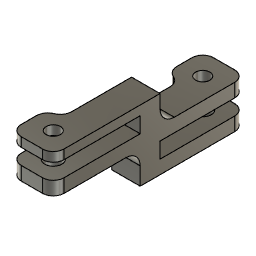
master v6 (Autodesk Fusion 360 archive; units mm, degrees)
design "Linkage"
Autodesk Fusion 360 part; units mm, degrees
sketch "Sketch1" plane through (0, 0, 0) normal (1, 0, 0) x (0, 1, 0)
  line L0 (-75.822, 4.0286) -> (-63.122, 4.0286)
  line L1 (-56.772, -1.661) -> (-41.532, -1.661)
  line L2 (-41.532, 5.959) -> (-53.8576, 5.959)
  line L3 (-60.2076, 10.8866) -> (-75.822, 10.8866)
  line L4 (-75.822, 4.0286) -> (-75.822, 6.4416)
  line L5 (-75.822, 6.4416) -> (-60.3127, 6.4416)
  line L6 (-60.3127, 6.4416) -> (-60.3127, 9.2356)
  line L7 (-60.3127, 9.2356) -> (-75.822, 9.2356)
  line L8 (-75.822, 9.2356) -> (-75.822, 10.8866)
  line L9 (-41.532, -1.661) -> (-41.532, 0.752)
  line L10 (-41.532, 0.752) -> (-56.772, 0.752)
  line L11 (-56.772, 0.752) -> (-56.772, 3.546)
  line L12 (-56.772, 3.546) -> (-41.532, 3.546)
  line L13 (-41.532, 3.546) -> (-41.532, 5.959)
  line L14 (-60.2076, 10.8866) -> (-56.772, 10.8866)
  line L15 (-56.772, 10.8866) -> (-56.772, 5.959)
  line L16 (-56.772, 5.959) -> (-53.8576, 5.959)
  line L17 (-56.772, -1.661) -> (-60.3127, -1.661)
  line L18 (-60.3127, -1.661) -> (-60.3127, 4.0286)
  line L19 (-60.3127, 4.0286) -> (-63.122, 4.0286)
  dimension "d2" = 7.62
  dimension "d3" = 6.858
  dimension "d4" = 12.7
  dimension "d5" = 15.24
  dimension "d9" = 2.413
  dimension "d10" = 15.24
  dimension "d12" = 6.35
  dimension "d35" = 15.5093
  dimension "d38" = 2.794
  dimension "d39" = 5.6896
  constraint horizontal L0
  constraint parallel L0 L1
  constraint perpendicular L0 L4
  constraint perpendicular L4 L5
  constraint perpendicular L5 L6
  constraint perpendicular L6 L7
  constraint perpendicular L3 L8
  constraint perpendicular L1 L9
  constraint perpendicular L9 L10
  constraint perpendicular L10 L11
  constraint perpendicular L11 L12
  constraint perpendicular L2 L13
  constraint equal L9 L13
  constraint equal L4 L9
  constraint collinear L9 L13
  constraint collinear L4 L8
  constraint parallel L12 L14
  constraint perpendicular L2 L15
  constraint perpendicular L15 L16
  constraint perpendicular L6 L17
  constraint perpendicular L17 L18
  constraint perpendicular L18 L19
  measures "d2" distance of L1 L2
  measures "d3" distance of L0 L3
  measures "d4" distance of L0.start L0.end
  measures "d5" distance of L1.start L1.end
  measures "d9" distance of L1.end L9.end
  measures "d10" distance of L9.end L10.end
  measures "d12" horizontal distance of L2.end L3.start
  measures "d35" distance of L4.end L5.end
  measures "d38" distance of L5.end L6.end
  measures "d39" distance of L5 L10
extrude "Extrude1" add sketch "Sketch1" along normal blind 7.62
sketch "Sketch2" plane through (0, 0, 6.4416) normal (0, 0, 1) x (-1, 0, 0)
  line L0 (0, 60.3127) -> (0, 75.822)
  line L1 (0, 75.822) -> (-7.62, 75.822)
  line L2 (-7.62, 75.822) -> (-7.62, 60.3127)
  line L3 (-7.62, 60.3127) -> (0, 60.3127)
  line L4 (-3.81, 75.822) -> (-3.81, 72.012) construction
  circle A0 centre (-3.81, 72.012) radius 1.27
  dimension "d15" = 3.81
  dimension "d16" = 2.54
  constraint midpoint L1 L4.start
  constraint perpendicular L1 L4
  constraint coincident L4.end A0.centre
  measures "d15" distance of L4.start L4.end
  measures "d16" diameter of A0
extrude "Extrude2" cut sketch "Sketch2" along normal blind 8.128 and the other way blind 3.048 contours A0
sketch "Sketch3" plane through (0, 0, 0.752) normal (0, 0, 1) x (-1, 0, 0)
  line L0 (0, 41.532) -> (0, 56.772)
  line L1 (0, 56.772) -> (-7.62, 56.772)
  line L2 (-7.62, 56.772) -> (-7.62, 41.532)
  line L3 (-7.62, 41.532) -> (0, 41.532)
  line L4 (-3.81, 41.532) -> (-3.81, 45.342) construction
  circle A0 centre (-3.81, 45.342) radius 1.27
  dimension "d21" = 2.54
  constraint midpoint L3 L4.start
  constraint perpendicular L3 L4
  constraint coincident L4.end A0.centre
  measures "d21" diameter of A0
extrude "Extrude3" cut sketch "Sketch3" along normal blind 5.588 and the other way blind 4.318 contours A0
fillet "Fillet1" radius 1.905 8 edges at (0, -41.532, 4.7525) (7.62, -41.532, 4.7525) (0, -41.532, -0.4545) (7.62, -41.532, -0.4545) (0, -75.822, 5.2351) (7.62, -75.822, 5.2351) (7.62, -75.822, 10.0611) (0, -75.822, 10.0611)
sketch "Sketch4" plane through (0, 0, 10.8866) normal (0, 0, 1) x (-1, 0, 0)
  arc A0 (0, 73.917) -> (-1.905, 75.822) centre (-1.905, 73.917) ccw
  line L0 (-1.905, 75.822) -> (-5.715, 75.822)
  arc A1 (-5.715, 75.822) -> (-7.62, 73.917) centre (-5.715, 73.917) ccw
  line L1 (-7.62, 73.917) -> (-7.62, 56.772)
  line L2 (0, 56.772) -> (0, 73.917)
  circle A2 centre (-3.81, 72.012) radius 1.27
  line L3 (0, 47.882) -> (-2.54, 47.882)
  line L4 (-2.54, 47.882) -> (-2.54, 69.472)
  line L5 (-2.54, 69.472) -> (0, 69.472)
  line L6 (0, 69.472) -> (0, 47.882)
  circle A3 centre (-3.81, 45.342) radius 1.27
  line L7 (0, 47.882) -> (0, 49.8938)
  line L8 (-7.62, 56.772) -> (0, 56.772)
  dimension "d28" = 2.54
  dimension "d29" = 2.54
  dimension "d30" = 2.54
  constraint horizontal L3
  constraint vertical L4
  constraint horizontal L5
  constraint vertical L6
  constraint perpendicular L3 L7
  measures "d28" distance of A2.centre L5
  measures "d29" distance of L3 A3.centre
  measures "d30" distance of L3.start L3.end
extrude "Extrude4" cut sketch "Sketch4" against normal blind 20.32 contours L2 L4 L5 L6 L8 | L3 L4 L6 L7 L8
fillet "Fillet2" radius 2.032 8 edges at (2.54, -47.882, -0.4545) (2.54, -47.882, 4.7525) (2.54, -69.472, 5.2351) (2.54, -69.472, 10.0611) (0, -69.472, 10.0611) (0, -69.472, 5.2351) (0, -47.882, 4.7525) (0, -47.882, -0.4545)
fillet "Fillet3" radius 2.54 2 edges at (5.08, -60.3127, 4.0286) (5.08, -56.772, 5.959)
sketch "Sketch5" plane through (0, 0, 4.0286) normal (0, 0, -1) x (1, 0, 0)
  line L0 (2.54, 62.8527) -> (7.62, 62.8527)
  line L1 (7.62, 62.8527) -> (7.62, 73.917)
  arc A0 (7.62, 73.917) -> (5.715, 75.822) centre (5.715, 73.917) ccw
  line L2 (5.715, 75.822) -> (1.905, 75.822)
  arc A1 (1.905, 75.822) -> (0, 73.917) centre (1.905, 73.917) ccw
  line L3 (0, 73.917) -> (0, 71.2075)
  arc A2 (0, 71.2075) -> (1.27, 69.3237) centre (2.032, 71.2075) ccw
  arc A3 (2.54, 67.44) -> (1.27, 69.3237) centre (0.508, 67.44) ccw
  line L4 (2.54, 67.44) -> (2.54, 62.8527)
  circle A4 centre (3.81, 72.012) radius 1.27
  circle A5 centre (3.81, 72.012) radius 1.524
  dimension "d40" = 3.048
  constraint concentric A4 A5
  measures "d40" diameter of A5
extrude "Extrude5" cut sketch "Sketch5" against normal blind 2.54 contours A5
sketch "Sketch6" plane through (0, 0, -1.661) normal (0, 0, -1) x (1, 0, 0)
  arc A0 (1.27, 48.0303) -> (0, 46.1466) centre (2.032, 46.1466) ccw
  line L0 (0, 46.1466) -> (0, 43.437)
  arc A1 (0, 43.437) -> (1.905, 41.532) centre (1.905, 43.437) ccw
  line L1 (1.905, 41.532) -> (5.715, 41.532)
  arc A2 (5.715, 41.532) -> (7.62, 43.437) centre (5.715, 43.437) ccw
  line L2 (7.62, 43.437) -> (7.62, 60.3127)
  line L3 (7.62, 60.3127) -> (2.54, 60.3127)
  line L4 (2.54, 60.3127) -> (2.54, 49.914)
  arc A3 (1.27, 48.0303) -> (2.54, 49.914) centre (0.508, 49.914) ccw
  circle A4 centre (3.81, 45.342) radius 1.27
  circle A5 centre (3.81, 45.342) radius 1.524
  dimension "d43" = 3.048
  constraint concentric A4 A5
  measures "d43" diameter of A5
extrude "Extrude6" cut sketch "Sketch6" against normal blind 2.54 contours A5
